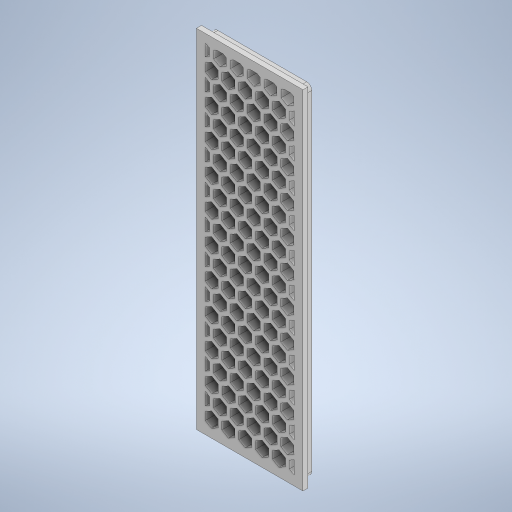
# Autodesk Inventor part: Ventilacion
Saved by Autodesk Inventor 2024 (Build 280153000, 153)
## iProperties
Created: 2023-11-28
Part Number: Ventilacion
Material: Genérico
Document SubType Name: Modeling
Designer: sergi
Density: 1 g/cm^3
Appearance: Valor por defecto
Author: sergi
Autodesk Inventor part; units mm, degrees
(part 1 of 2)
ref_plane "YZ Plane" through (0, 0, 0) normal (1, 0, 0) x (0, 1, 0)
ref_plane "XZ Plane" through (0, 0, 0) normal (0, 1, 0) x (-1, 0, 0)
ref_plane "XY Plane" through (0, 0, 0) normal (0, 0, 1) x (1, 0, 0)
sketch "Boceto1" plane through (0, 0, 0) normal (0, 0, 1) x (1, 0, 0)
  line L0 (-1, 144.7) -> (-1, 9) projected
  line L1 (-1, 9) -> (-41, 9) projected
  line L2 (-41, 9) -> (-41, 144.7) projected
  line L3 (-41, 144.7) -> (-1, 144.7) projected
  line L4 (8, 153.7) -> (-50, 153.7) projected
  line L5 (-50, 0) -> (-50, 153.7) projected
  line L6 (8, 0) -> (-50, 0) projected
  line L7 (8, 153.7) -> (8, 0) projected
  line L8 (-41, 9) -> (-1, 9)
  line L9 (-1, 9) -> (-1, 144.7)
  line L10 (-1, 144.7) -> (-41, 144.7)
  line L11 (-41, 144.7) -> (-41, 9)
  line L12 (-40.65, 144.35) -> (-40.65, 9.35)
  line L13 (-40.65, 9.35) -> (-1.35, 9.35)
  line L14 (-1.35, 9.35) -> (-1.35, 144.35)
  line L15 (-1.35, 144.35) -> (-40.65, 144.35)
  line L16 (-3.35, 11.35) -> (-38.65, 11.35)
  line L17 (-38.65, 11.35) -> (-38.65, 142.35)
  line L18 (-38.65, 142.35) -> (-3.35, 142.35)
  line L19 (-3.35, 142.35) -> (-3.35, 11.35)
  line L20 (-36.1519, 17.25) -> (-33.5538, 15.75)
  line L21 (-33.5538, 15.75) -> (-33.5538, 12.75)
  line L22 (-33.5538, 12.75) -> (-36.1519, 11.25)
  line L23 (-36.1519, 11.25) -> (-38.75, 12.75)
  line L24 (-38.75, 12.75) -> (-38.75, 15.75)
  line L25 (-38.75, 15.75) -> (-36.1519, 17.25)
  line L26 (-38.65, 11.35) -> (-38.65, 12.75)
  line L27 (-30.2058, 21.75) -> (-30.2058, 18.75)
  line L28 (-30.2058, 18.75) -> (-32.8038, 17.25)
  line L29 (-32.8038, 17.25) -> (-35.4019, 18.75)
  line L30 (-35.4019, 18.75) -> (-35.4019, 21.75)
  line L31 (-35.4019, 21.75) -> (-32.8038, 23.25)
  line L32 (-32.8038, 23.25) -> (-30.2058, 21.75)
  line L33 (-26.8577, 15.75) -> (-26.8577, 12.75)
  line L34 (-26.8577, 12.75) -> (-29.4558, 11.25)
  line L35 (-29.4558, 11.25) -> (-32.0538, 12.75)
  line L36 (-32.0538, 12.75) -> (-32.0538, 15.75)
  line L37 (-32.0538, 15.75) -> (-29.4558, 17.25)
  line L38 (-29.4558, 17.25) -> (-26.8577, 15.75)
  line L39 (-28.7058, 18.75) -> (-28.7058, 21.75)
  line L40 (-28.7058, 21.75) -> (-26.1077, 23.25)
  line L41 (-26.1077, 23.25) -> (-23.5096, 21.75)
  line L42 (-23.5096, 21.75) -> (-23.5096, 18.75)
  line L43 (-23.5096, 18.75) -> (-26.1077, 17.25)
  line L44 (-26.1077, 17.25) -> (-28.7058, 18.75)
  line L45 (-22.0096, 18.75) -> (-22.0096, 21.75)
  line L46 (-22.0096, 21.75) -> (-19.4115, 23.25)
  line L47 (-19.4115, 23.25) -> (-16.8135, 21.75)
  line L48 (-16.8135, 21.75) -> (-16.8135, 18.75)
  line L49 (-16.8135, 18.75) -> (-19.4115, 17.25)
  line L50 (-19.4115, 17.25) -> (-22.0096, 18.75)
  line L51 (-15.3135, 18.75) -> (-15.3135, 21.75)
  line L52 (-15.3135, 21.75) -> (-12.7154, 23.25)
  line L53 (-12.7154, 23.25) -> (-10.1173, 21.75)
  line L54 (-10.1173, 21.75) -> (-10.1173, 18.75)
  line L55 (-10.1173, 18.75) -> (-12.7154, 17.25)
  line L56 (-12.7154, 17.25) -> (-15.3135, 18.75)
  line L57 (-8.6173, 18.75) -> (-8.6173, 21.75)
  line L58 (-8.6173, 21.75) -> (-6.0192, 23.25)
  line L59 (-6.0192, 23.25) -> (-3.4212, 21.75)
  line L60 (-3.4212, 21.75) -> (-3.4212, 18.75)
  line L61 (-3.4212, 18.75) -> (-6.0192, 17.25)
  line L62 (-6.0192, 17.25) -> (-8.6173, 18.75)
  line L63 (-40.65, 17.914) -> (-42.0981, 18.75)
  line L64 (-36.9019, 21.75) -> (-36.9019, 18.75)
  line L65 (-42.0981, 18.75) -> (-42.0981, 21.75)
  line L66 (-42.0981, 21.75) -> (-39.5, 23.25)
  line L67 (-38.65, 22.7593) -> (-36.9019, 21.75)
  line L68 (-36.9019, 18.75) -> (-39.5, 17.25)
  line L69 (-30.2058, 33.6998) -> (-30.2058, 30.6998)
  line L70 (-30.2058, 30.6998) -> (-32.8038, 29.1998)
  line L71 (-32.8038, 29.1998) -> (-35.4019, 30.6998)
  line L72 (-35.4019, 30.6998) -> (-35.4019, 33.6998)
  line L73 (-35.4019, 33.6998) -> (-32.8038, 35.1998)
  line L74 (-32.8038, 35.1998) -> (-30.2058, 33.6998)
  line L75 (-28.7058, 30.6998) -> (-28.7058, 33.6998)
  line L76 (-28.7058, 33.6998) -> (-26.1077, 35.1998)
  line L77 (-26.1077, 35.1998) -> (-23.5096, 33.6998)
  line L78 (-23.5096, 33.6998) -> (-23.5096, 30.6998)
  line L79 (-23.5096, 30.6998) -> (-26.1077, 29.1998)
  line L80 (-26.1077, 29.1998) -> (-28.7058, 30.6998)
  line L81 (-19.4115, 29.1998) -> (-22.0096, 30.6998)
  line L82 (-16.8135, 33.6998) -> (-16.8135, 30.6998)
  line L83 (-22.0096, 30.6998) -> (-22.0096, 33.6998)
  line L84 (-22.0096, 33.6998) -> (-19.4115, 35.1998)
  line L85 (-19.4115, 35.1998) -> (-16.8135, 33.6998)
  line L86 (-16.8135, 30.6998) -> (-19.4115, 29.1998)
  line L87 (-12.7154, 29.1998) -> (-15.3135, 30.6998)
  line L88 (-10.1173, 33.6998) -> (-10.1173, 30.6998)
  line L89 (-15.3135, 30.6998) -> (-15.3135, 33.6998)
  line L90 (-15.3135, 33.6998) -> (-12.7154, 35.1998)
  line L91 (-12.7154, 35.1998) -> (-10.1173, 33.6998)
  line L92 (-10.1173, 30.6998) -> (-12.7154, 29.1998)
  line L93 (-6.0192, 29.1998) -> (-8.6173, 30.6998)
  line L94 (-3.4212, 33.6998) -> (-3.4212, 30.6998)
  line L95 (-8.6173, 30.6998) -> (-8.6173, 33.6998)
  line L96 (-8.6173, 33.6998) -> (-6.0192, 35.1998)
  line L97 (-6.0192, 35.1998) -> (-3.4212, 33.6998)
  line L98 (-3.4212, 30.6998) -> (-6.0192, 29.1998)
  line L99 (-42.0981, 30.6998) -> (-42.0981, 33.6998)
  line L100 (-42.0981, 33.6998) -> (-39.5, 35.1998)
  line L101 (-39.5, 29.1998) -> (-42.0981, 30.6998)
  line L102 (-36.9019, 33.6998) -> (-36.9019, 30.6998)
  line L103 (-38.65, 34.709) -> (-36.9019, 33.6998)
  line L104 (-36.9019, 30.6998) -> (-38.65, 29.6905)
  line L105 (-26.8577, 39.6998) -> (-26.8577, 36.6998)
  line L106 (-26.8577, 36.6998) -> (-29.4558, 35.1998)
  line L107 (-29.4558, 35.1998) -> (-32.0538, 36.6998)
  line L108 (-32.0538, 36.6998) -> (-32.0538, 39.6998)
  line L109 (-32.0538, 39.6998) -> (-29.4558, 41.1998)
  line L110 (-29.4558, 41.1998) -> (-26.8577, 39.6998)
  line L111 (-25.3577, 36.6998) -> (-25.3577, 39.6998)
  line L112 (-25.3577, 39.6998) -> (-22.7596, 41.1998)
  line L113 (-22.7596, 41.1998) -> (-20.1615, 39.6998)
  line L114 (-20.1615, 39.6998) -> (-20.1615, 36.6998)
  line L115 (-20.1615, 36.6998) -> (-22.7596, 35.1998)
  line L116 (-22.7596, 35.1998) -> (-25.3577, 36.6998)
  line L117 (-16.0635, 35.1998) -> (-18.6615, 36.6998)
  line L118 (-13.4654, 39.6998) -> (-13.4654, 36.6998)
  line L119 (-18.6615, 36.6998) -> (-18.6615, 39.6998)
  line L120 (-18.6615, 39.6998) -> (-16.0635, 41.1998)
  line L121 (-16.0635, 41.1998) -> (-13.4654, 39.6998)
  line L122 (-13.4654, 36.6998) -> (-16.0635, 35.1998)
  line L123 (-9.3673, 35.1998) -> (-11.9654, 36.6998)
  line L124 (-6.7692, 39.6998) -> (-6.7692, 36.6998)
  line L125 (-11.9654, 36.6998) -> (-11.9654, 39.6998)
  line L126 (-11.9654, 39.6998) -> (-9.3673, 41.1998)
  line L127 (-9.3673, 41.1998) -> (-6.7692, 39.6998)
  line L128 (-6.7692, 36.6998) -> (-9.3673, 35.1998)
  line L129 (-2.6712, 35.1998) -> (-5.2692, 36.6998)
  line L130 (-0.0731, 39.6998) -> (-0.0731, 36.6998)
  line L131 (-5.2692, 36.6998) -> (-5.2692, 39.6998)
  line L132 (-5.2692, 39.6998) -> (-2.6712, 41.1998)
  line L133 (-1.35, 40.437) -> (-0.0731, 39.6998)
  line L134 (-0.0731, 36.6998) -> (-1.35, 35.9625)
  line L135 (-38.75, 36.6998) -> (-38.75, 39.6998)
  line L136 (-38.75, 39.6998) -> (-36.1519, 41.1998)
  line L137 (-36.1519, 35.1998) -> (-38.75, 36.6998)
  line L138 (-33.5538, 39.6998) -> (-33.5538, 36.6998)
  line L139 (-36.1519, 41.1998) -> (-33.5538, 39.6998)
  line L140 (-33.5538, 36.6998) -> (-36.1519, 35.1998)
  line L141 (-30.2058, 45.6998) -> (-30.2058, 42.6998)
  line L142 (-30.2058, 42.6998) -> (-32.8038, 41.1998)
  line L143 (-32.8038, 41.1998) -> (-35.4019, 42.6998)
  line L144 (-35.4019, 42.6998) -> (-35.4019, 45.6998)
  line L145 (-35.4019, 45.6998) -> (-32.8038, 47.1998)
  line L146 (-32.8038, 47.1998) -> (-30.2058, 45.6998)
  line L147 (-28.7058, 42.6998) -> (-28.7058, 45.6998)
  line L148 (-28.7058, 45.6998) -> (-26.1077, 47.1998)
  line L149 (-26.1077, 47.1998) -> (-23.5096, 45.6998)
  line L150 (-23.5096, 45.6998) -> (-23.5096, 42.6998)
  line L151 (-23.5096, 42.6998) -> (-26.1077, 41.1998)
  line L152 (-26.1077, 41.1998) -> (-28.7058, 42.6998)
  line L153 (-19.4115, 41.1998) -> (-22.0096, 42.6998)
  line L154 (-16.8135, 45.6998) -> (-16.8135, 42.6998)
  line L155 (-22.0096, 42.6998) -> (-22.0096, 45.6998)
  line L156 (-22.0096, 45.6998) -> (-19.4115, 47.1998)
  line L157 (-19.4115, 47.1998) -> (-16.8135, 45.6998)
  line L158 (-16.8135, 42.6998) -> (-19.4115, 41.1998)
  line L159 (-12.7154, 41.1998) -> (-15.3135, 42.6998)
  line L160 (-10.1173, 45.6998) -> (-10.1173, 42.6998)
  line L161 (-15.3135, 42.6998) -> (-15.3135, 45.6998)
  line L162 (-15.3135, 45.6998) -> (-12.7154, 47.1998)
  line L163 (-12.7154, 47.1998) -> (-10.1173, 45.6998)
  line L164 (-10.1173, 42.6998) -> (-12.7154, 41.1998)
  line L165 (-6.0192, 41.1998) -> (-8.6173, 42.6998)
  line L166 (-3.4212, 45.6998) -> (-3.4212, 42.6998)
  line L167 (-8.6173, 42.6998) -> (-8.6173, 45.6998)
  line L168 (-8.6173, 45.6998) -> (-6.0192, 47.1998)
  line L169 (-6.0192, 47.1998) -> (-3.4212, 45.6998)
  line L170 (-3.4212, 42.6998) -> (-6.0192, 41.1998)
  line L171 (-42.0981, 42.6998) -> (-42.0981, 45.6998)
  line L172 (-42.0981, 45.6998) -> (-40.65, 46.5358)
  line L173 (-40.65, 41.8637) -> (-42.0981, 42.6998)
  line L174 (-36.9019, 45.6998) -> (-36.9019, 42.6998)
  line L175 (-39.5, 47.1998) -> (-36.9019, 45.6998)
  line L176 (-36.9019, 42.6998) -> (-39.5, 41.1998)
  line L177 (-26.8577, 51.6998) -> (-26.8577, 48.6998)
  line L178 (-26.8577, 48.6998) -> (-29.4558, 47.1998)
  line L179 (-29.4558, 47.1998) -> (-32.0538, 48.6998)
  line L180 (-32.0538, 48.6998) -> (-32.0538, 51.6998)
  line L181 (-32.0538, 51.6998) -> (-29.4558, 53.1998)
  line L182 (-29.4558, 53.1998) -> (-26.8577, 51.6998)
  line L183 (-25.3577, 48.6998) -> (-25.3577, 51.6998)
  line L184 (-25.3577, 51.6998) -> (-22.7596, 53.1998)
  line L185 (-22.7596, 53.1998) -> (-20.1615, 51.6998)
  line L186 (-20.1615, 51.6998) -> (-20.1615, 48.6998)
  line L187 (-20.1615, 48.6998) -> (-22.7596, 47.1998)
  line L188 (-22.7596, 47.1998) -> (-25.3577, 48.6998)
  line L189 (-16.0635, 47.1998) -> (-18.6615, 48.6998)
  line L190 (-13.4654, 51.6998) -> (-13.4654, 48.6998)
  line L191 (-18.6615, 48.6998) -> (-18.6615, 51.6998)
  line L192 (-18.6615, 51.6998) -> (-16.0635, 53.1998)
  line L193 (-16.0635, 53.1998) -> (-13.4654, 51.6998)
  line L194 (-13.4654, 48.6998) -> (-16.0635, 47.1998)
  line L195 (-9.3673, 47.1998) -> (-11.9654, 48.6998)
  line L196 (-6.7692, 51.6998) -> (-6.7692, 48.6998)
  line L197 (-11.9654, 48.6998) -> (-11.9654, 51.6998)
  line L198 (-11.9654, 51.6998) -> (-9.3673, 53.1998)
  line L199 (-9.3673, 53.1998) -> (-6.7692, 51.6998)
  line L200 (-6.7692, 48.6998) -> (-9.3673, 47.1998)
  line L201 (-2.6712, 47.1998) -> (-5.2692, 48.6998)
  line L202 (-0.0731, 51.6998) -> (-0.0731, 48.6998)
  line L203 (-5.2692, 48.6998) -> (-5.2692, 51.6998)
  line L204 (-5.2692, 51.6998) -> (-2.6712, 53.1998)
  line L205 (-1.35, 52.437) -> (-0.0731, 51.6998)
  line L206 (-0.0731, 48.6998) -> (-1.35, 47.9625)
  line L207 (-38.75, 48.6998) -> (-38.75, 51.6998)
  line L208 (-38.75, 51.6998) -> (-36.1519, 53.1998)
  line L209 (-36.1519, 47.1998) -> (-38.75, 48.6998)
  line L210 (-33.5538, 51.6998) -> (-33.5538, 48.6998)
  line L211 (-36.1519, 53.1998) -> (-33.5538, 51.6998)
  line L212 (-33.5538, 48.6998) -> (-36.1519, 47.1998)
  line L213 (-30.2058, 57.6998) -> (-30.2058, 54.6998)
  line L214 (-30.2058, 54.6998) -> (-32.8038, 53.1998)
  line L215 (-32.8038, 53.1998) -> (-35.4019, 54.6998)
  line L216 (-35.4019, 54.6998) -> (-35.4019, 57.6998)
  line L217 (-35.4019, 57.6998) -> (-32.8038, 59.1998)
  line L218 (-32.8038, 59.1998) -> (-30.2058, 57.6998)
  line L219 (-28.7058, 54.6998) -> (-28.7058, 57.6998)
  line L220 (-28.7058, 57.6998) -> (-26.1077, 59.1998)
  line L221 (-26.1077, 59.1998) -> (-23.5096, 57.6998)
  line L222 (-23.5096, 57.6998) -> (-23.5096, 54.6998)
  line L223 (-23.5096, 54.6998) -> (-26.1077, 53.1998)
  line L224 (-26.1077, 53.1998) -> (-28.7058, 54.6998)
  line L225 (-19.4115, 53.1998) -> (-22.0096, 54.6998)
  line L226 (-16.8135, 57.6998) -> (-16.8135, 54.6998)
  line L227 (-22.0096, 54.6998) -> (-22.0096, 57.6998)
  line L228 (-22.0096, 57.6998) -> (-19.4115, 59.1998)
  line L229 (-19.4115, 59.1998) -> (-16.8135, 57.6998)
  line L230 (-16.8135, 54.6998) -> (-19.4115, 53.1998)
  line L231 (-12.7154, 53.1998) -> (-15.3135, 54.6998)
  line L232 (-10.1173, 57.6998) -> (-10.1173, 54.6998)
  line L233 (-15.3135, 54.6998) -> (-15.3135, 57.6998)
  line L234 (-15.3135, 57.6998) -> (-12.7154, 59.1998)
  line L235 (-12.7154, 59.1998) -> (-10.1173, 57.6998)
  line L236 (-10.1173, 54.6998) -> (-12.7154, 53.1998)
  line L237 (-6.0192, 53.1998) -> (-8.6173, 54.6998)
  line L238 (-3.4212, 57.6998) -> (-3.4212, 54.6998)
  line L239 (-8.6173, 54.6998) -> (-8.6173, 57.6998)
  line L240 (-8.6173, 57.6998) -> (-6.0192, 59.1998)
  line L241 (-6.0192, 59.1998) -> (-3.4212, 57.6998)
  line L242 (-3.4212, 54.6998) -> (-6.0192, 53.1998)
  line L243 (-42.0981, 54.6998) -> (-42.0981, 57.6998)
  line L244 (-42.0981, 57.6998) -> (-40.65, 58.5358)
  line L245 (-40.65, 53.8637) -> (-42.0981, 54.6998)
  line L246 (-36.9019, 57.6998) -> (-36.9019, 54.6998)
  line L247 (-39.5, 59.1998) -> (-36.9019, 57.6998)
  line L248 (-36.9019, 54.6998) -> (-39.5, 53.1998)
  line L249 (-26.8577, 63.6998) -> (-26.8577, 60.6998)
  line L250 (-26.8577, 60.6998) -> (-29.4558, 59.1998)
  line L251 (-29.4558, 59.1998) -> (-32.0538, 60.6998)
  line L252 (-32.0538, 60.6998) -> (-32.0538, 63.6998)
  line L253 (-32.0538, 63.6998) -> (-29.4558, 65.1998)
  line L254 (-29.4558, 65.1998) -> (-26.8577, 63.6998)
  line L255 (-25.3577, 60.6998) -> (-25.3577, 63.6998)
  line L256 (-25.3577, 63.6998) -> (-22.7596, 65.1998)
  line L257 (-22.7596, 65.1998) -> (-20.1615, 63.6998)
  line L258 (-20.1615, 63.6998) -> (-20.1615, 60.6998)
  line L259 (-20.1615, 60.6998) -> (-22.7596, 59.1998)
  line L260 (-22.7596, 59.1998) -> (-25.3577, 60.6998)
  line L261 (-16.0635, 59.1998) -> (-18.6615, 60.6998)
  line L262 (-13.4654, 63.6998) -> (-13.4654, 60.6998)
  line L263 (-18.6615, 60.6998) -> (-18.6615, 63.6998)
  line L264 (-18.6615, 63.6998) -> (-16.0635, 65.1998)
  line L265 (-16.0635, 65.1998) -> (-13.4654, 63.6998)
  line L266 (-13.4654, 60.6998) -> (-16.0635, 59.1998)
  line L267 (-9.3673, 59.1998) -> (-11.9654, 60.6998)
  line L268 (-6.7692, 63.6998) -> (-6.7692, 60.6998)
  line L269 (-11.9654, 60.6998) -> (-11.9654, 63.6998)
  line L270 (-11.9654, 63.6998) -> (-9.3673, 65.1998)
  line L271 (-9.3673, 65.1998) -> (-6.7692, 63.6998)
  line L272 (-6.7692, 60.6998) -> (-9.3673, 59.1998)
  line L273 (-2.6712, 59.1998) -> (-5.2692, 60.6998)
  line L274 (-0.0731, 63.6998) -> (-0.0731, 60.6998)
  line L275 (-5.2692, 60.6998) -> (-5.2692, 63.6998)
  line L276 (-5.2692, 63.6998) -> (-2.6712, 65.1998)
  line L277 (-1.35, 64.437) -> (-0.0731, 63.6998)
  line L278 (-0.0731, 60.6998) -> (-1.35, 59.9625)
  line L279 (-38.75, 60.6998) -> (-38.75, 63.6998)
  line L280 (-38.75, 63.6998) -> (-36.1519, 65.1998)
  line L281 (-36.1519, 59.1998) -> (-38.75, 60.6998)
  line L282 (-33.5538, 63.6998) -> (-33.5538, 60.6998)
  line L283 (-36.1519, 65.1998) -> (-33.5538, 63.6998)
  line L284 (-33.5538, 60.6998) -> (-36.1519, 59.1998)
  line L285 (-30.2058, 69.6998) -> (-30.2058, 66.6998)
  line L286 (-30.2058, 66.6998) -> (-32.8038, 65.1998)
  line L287 (-32.8038, 65.1998) -> (-35.4019, 66.6998)
  line L288 (-35.4019, 66.6998) -> (-35.4019, 69.6998)
  line L289 (-35.4019, 69.6998) -> (-32.8038, 71.1998)
  line L290 (-32.8038, 71.1998) -> (-30.2058, 69.6998)
  line L291 (-28.7058, 66.6998) -> (-28.7058, 69.6998)
  line L292 (-28.7058, 69.6998) -> (-26.1077, 71.1998)
  line L293 (-26.1077, 71.1998) -> (-23.5096, 69.6998)
  line L294 (-23.5096, 69.6998) -> (-23.5096, 66.6998)
  line L295 (-23.5096, 66.6998) -> (-26.1077, 65.1998)
  line L296 (-26.1077, 65.1998) -> (-28.7058, 66.6998)
  line L297 (-19.4115, 65.1998) -> (-22.0096, 66.6998)
  line L298 (-16.8135, 69.6998) -> (-16.8135, 66.6998)
  line L299 (-22.0096, 66.6998) -> (-22.0096, 69.6998)
  line L300 (-22.0096, 69.6998) -> (-19.4115, 71.1998)
  line L301 (-19.4115, 71.1998) -> (-16.8135, 69.6998)
  line L302 (-16.8135, 66.6998) -> (-19.4115, 65.1998)
  line L303 (-12.7154, 65.1998) -> (-15.3135, 66.6998)
  line L304 (-10.1173, 69.6998) -> (-10.1173, 66.6998)
  line L305 (-15.3135, 66.6998) -> (-15.3135, 69.6998)
  line L306 (-15.3135, 69.6998) -> (-12.7154, 71.1998)
  line L307 (-12.7154, 71.1998) -> (-10.1173, 69.6998)
  line L308 (-10.1173, 66.6998) -> (-12.7154, 65.1998)
  line L309 (-6.0192, 65.1998) -> (-8.6173, 66.6998)
  line L310 (-3.4212, 69.6998) -> (-3.4212, 66.6998)
  line L311 (-8.6173, 66.6998) -> (-8.6173, 69.6998)
  line L312 (-8.6173, 69.6998) -> (-6.0192, 71.1998)
  line L313 (-6.0192, 71.1998) -> (-3.4212, 69.6998)
  line L314 (-3.4212, 66.6998) -> (-6.0192, 65.1998)
  line L315 (-42.0981, 66.6998) -> (-42.0981, 69.6998)
  line L316 (-42.0981, 69.6998) -> (-40.65, 70.5358)
  line L317 (-40.65, 65.8637) -> (-42.0981, 66.6998)
  line L318 (-36.9019, 69.6998) -> (-36.9019, 66.6998)
  line L319 (-39.5, 71.1998) -> (-36.9019, 69.6998)
  line L320 (-36.9019, 66.6998) -> (-39.5, 65.1998)
  line L321 (-26.8577, 75.6998) -> (-26.8577, 72.6998)
  line L322 (-26.8577, 72.6998) -> (-29.4558, 71.1998)
  line L323 (-29.4558, 71.1998) -> (-32.0538, 72.6998)
  line L324 (-32.0538, 72.6998) -> (-32.0538, 75.6998)
  line L325 (-32.0538, 75.6998) -> (-29.4558, 77.1998)
  line L326 (-29.4558, 77.1998) -> (-26.8577, 75.6998)
  line L327 (-25.3577, 72.6998) -> (-25.3577, 75.6998)
  line L328 (-25.3577, 75.6998) -> (-22.7596, 77.1998)
  line L329 (-22.7596, 77.1998) -> (-20.1615, 75.6998)
  line L330 (-20.1615, 75.6998) -> (-20.1615, 72.6998)
  line L331 (-20.1615, 72.6998) -> (-22.7596, 71.1998)
  line L332 (-22.7596, 71.1998) -> (-25.3577, 72.6998)
  line L333 (-16.0635, 71.1998) -> (-18.6615, 72.6998)
  line L334 (-13.4654, 75.6998) -> (-13.4654, 72.6998)
  line L335 (-18.6615, 72.6998) -> (-18.6615, 75.6998)
  line L336 (-18.6615, 75.6998) -> (-16.0635, 77.1998)
  line L337 (-16.0635, 77.1998) -> (-13.4654, 75.6998)
  line L338 (-13.4654, 72.6998) -> (-16.0635, 71.1998)
  line L339 (-9.3673, 71.1998) -> (-11.9654, 72.6998)
  line L340 (-6.7692, 75.6998) -> (-6.7692, 72.6998)
  line L341 (-11.9654, 72.6998) -> (-11.9654, 75.6998)
  line L342 (-11.9654, 75.6998) -> (-9.3673, 77.1998)
  line L343 (-9.3673, 77.1998) -> (-6.7692, 75.6998)
  line L344 (-6.7692, 72.6998) -> (-9.3673, 71.1998)
  line L345 (-2.6712, 71.1998) -> (-5.2692, 72.6998)
  line L346 (-0.0731, 75.6998) -> (-0.0731, 72.6998)
  line L347 (-5.2692, 72.6998) -> (-5.2692, 75.6998)
  line L348 (-5.2692, 75.6998) -> (-2.6712, 77.1998)
  line L349 (-1.35, 76.437) -> (-0.0731, 75.6998)
  line L350 (-0.0731, 72.6998) -> (-1.35, 71.9625)
  line L351 (-38.75, 72.6998) -> (-38.75, 75.6998)
  line L352 (-38.75, 75.6998) -> (-36.1519, 77.1998)
  line L353 (-36.1519, 71.1998) -> (-38.75, 72.6998)
  line L354 (-33.5538, 75.6998) -> (-33.5538, 72.6998)
  line L355 (-36.1519, 77.1998) -> (-33.5538, 75.6998)
  line L356 (-33.5538, 72.6998) -> (-36.1519, 71.1998)
  line L357 (-30.2058, 81.6998) -> (-30.2058, 78.6998)
  line L358 (-30.2058, 78.6998) -> (-32.8038, 77.1998)
  line L359 (-32.8038, 77.1998) -> (-35.4019, 78.6998)
  line L360 (-35.4019, 78.6998) -> (-35.4019, 81.6998)
  line L361 (-35.4019, 81.6998) -> (-32.8038, 83.1998)
  line L362 (-32.8038, 83.1998) -> (-30.2058, 81.6998)
  line L363 (-28.7058, 78.6998) -> (-28.7058, 81.6998)
  line L364 (-28.7058, 81.6998) -> (-26.1077, 83.1998)
  line L365 (-26.1077, 83.1998) -> (-23.5096, 81.6998)
  line L366 (-23.5096, 81.6998) -> (-23.5096, 78.6998)
  line L367 (-23.5096, 78.6998) -> (-26.1077, 77.1998)
  line L368 (-26.1077, 77.1998) -> (-28.7058, 78.6998)
  line L369 (-19.4115, 77.1998) -> (-22.0096, 78.6998)
  line L370 (-16.8135, 81.6998) -> (-16.8135, 78.6998)
  line L371 (-22.0096, 78.6998) -> (-22.0096, 81.6998)
  line L372 (-22.0096, 81.6998) -> (-19.4115, 83.1998)
  line L373 (-19.4115, 83.1998) -> (-16.8135, 81.6998)
  line L374 (-16.8135, 78.6998) -> (-19.4115, 77.1998)
  line L375 (-12.7154, 77.1998) -> (-15.3135, 78.6998)
  line L376 (-10.1173, 81.6998) -> (-10.1173, 78.6998)
  line L377 (-15.3135, 78.6998) -> (-15.3135, 81.6998)
  line L378 (-15.3135, 81.6998) -> (-12.7154, 83.1998)
  line L379 (-12.7154, 83.1998) -> (-10.1173, 81.6998)
  line L380 (-10.1173, 78.6998) -> (-12.7154, 77.1998)
  line L381 (-6.0192, 77.1998) -> (-8.6173, 78.6998)
  line L382 (-3.4212, 81.6998) -> (-3.4212, 78.6998)
  line L383 (-8.6173, 78.6998) -> (-8.6173, 81.6998)
  line L384 (-8.6173, 81.6998) -> (-6.0192, 83.1998)
  line L385 (-6.0192, 83.1998) -> (-3.4212, 81.6998)
  line L386 (-3.4212, 78.6998) -> (-6.0192, 77.1998)
  line L387 (-42.0981, 78.6998) -> (-42.0981, 81.6998)
  line L388 (-42.0981, 81.6998) -> (-40.65, 82.5358)
  line L389 (-40.65, 77.8637) -> (-42.0981, 78.6998)
  line L390 (-36.9019, 81.6998) -> (-36.9019, 78.6998)
  line L391 (-39.5, 83.1998) -> (-36.9019, 81.6998)
  line L392 (-36.9019, 78.6998) -> (-39.5, 77.1998)
  line L393 (-26.8577, 87.6998) -> (-26.8577, 84.6998)
  line L394 (-26.8577, 84.6998) -> (-29.4558, 83.1998)
  line L395 (-29.4558, 83.1998) -> (-32.0538, 84.6998)
  line L396 (-32.0538, 84.6998) -> (-32.0538, 87.6998)
  line L397 (-32.0538, 87.6998) -> (-29.4558, 89.1998)
  line L398 (-29.4558, 89.1998) -> (-26.8577, 87.6998)
  line L399 (-25.3577, 84.6998) -> (-25.3577, 87.6998)
  line L400 (-25.3577, 87.6998) -> (-22.7596, 89.1998)
  line L401 (-22.7596, 89.1998) -> (-20.1615, 87.6998)
  line L402 (-20.1615, 87.6998) -> (-20.1615, 84.6998)
  line L403 (-20.1615, 84.6998) -> (-22.7596, 83.1998)
  line L404 (-22.7596, 83.1998) -> (-25.3577, 84.6998)
  line L405 (-16.0635, 83.1998) -> (-18.6615, 84.6998)
  line L406 (-13.4654, 87.6998) -> (-13.4654, 84.6998)
  line L407 (-18.6615, 84.6998) -> (-18.6615, 87.6998)
  line L408 (-18.6615, 87.6998) -> (-16.0635, 89.1998)
  line L409 (-16.0635, 89.1998) -> (-13.4654, 87.6998)
  line L410 (-13.4654, 84.6998) -> (-16.0635, 83.1998)
  line L411 (-9.3673, 83.1998) -> (-11.9654, 84.6998)
  line L412 (-6.7692, 87.6998) -> (-6.7692, 84.6998)
  line L413 (-11.9654, 84.6998) -> (-11.9654, 87.6998)
  line L414 (-11.9654, 87.6998) -> (-9.3673, 89.1998)
  line L415 (-9.3673, 89.1998) -> (-6.7692, 87.6998)
  line L416 (-6.7692, 84.6998) -> (-9.3673, 83.1998)
  line L417 (-2.6712, 83.1998) -> (-5.2692, 84.6998)
  line L418 (-0.0731, 87.6998) -> (-0.0731, 84.6998)
  line L419 (-5.2692, 84.6998) -> (-5.2692, 87.6998)
  line L420 (-5.2692, 87.6998) -> (-2.6712, 89.1998)
  line L421 (-1.35, 88.437) -> (-0.0731, 87.6998)
  line L422 (-0.0731, 84.6998) -> (-1.35, 83.9625)
  line L423 (-38.75, 84.6998) -> (-38.75, 87.6998)
  line L424 (-38.75, 87.6998) -> (-36.1519, 89.1998)
  line L425 (-36.1519, 83.1998) -> (-38.75, 84.6998)
  line L426 (-33.5538, 87.6998) -> (-33.5538, 84.6998)
  line L427 (-36.1519, 89.1998) -> (-33.5538, 87.6998)
  line L428 (-33.5538, 84.6998) -> (-36.1519, 83.1998)
  line L429 (-30.2058, 93.6998) -> (-30.2058, 90.6998)
  line L430 (-30.2058, 90.6998) -> (-32.8038, 89.1998)
  line L431 (-32.8038, 89.1998) -> (-35.4019, 90.6998)
  line L432 (-35.4019, 90.6998) -> (-35.4019, 93.6998)
  line L433 (-35.4019, 93.6998) -> (-32.8038, 95.1998)
  line L434 (-32.8038, 95.1998) -> (-30.2058, 93.6998)
  line L435 (-28.7058, 90.6998) -> (-28.7058, 93.6998)
  line L436 (-28.7058, 93.6998) -> (-26.1077, 95.1998)
  line L437 (-26.1077, 95.1998) -> (-23.5096, 93.6998)
  line L438 (-23.5096, 93.6998) -> (-23.5096, 90.6998)
  line L439 (-23.5096, 90.6998) -> (-26.1077, 89.1998)
  line L440 (-26.1077, 89.1998) -> (-28.7058, 90.6998)
  line L441 (-19.4115, 89.1998) -> (-22.0096, 90.6998)
  line L442 (-16.8135, 93.6998) -> (-16.8135, 90.6998)
  line L443 (-22.0096, 90.6998) -> (-22.0096, 93.6998)
  line L444 (-22.0096, 93.6998) -> (-19.4115, 95.1998)
  line L445 (-19.4115, 95.1998) -> (-16.8135, 93.6998)
  line L446 (-16.8135, 90.6998) -> (-19.4115, 89.1998)
  line L447 (-12.7154, 89.1998) -> (-15.3135, 90.6998)
  line L448 (-10.1173, 93.6998) -> (-10.1173, 90.6998)
  line L449 (-15.3135, 90.6998) -> (-15.3135, 93.6998)
  line L450 (-15.3135, 93.6998) -> (-12.7154, 95.1998)
  line L451 (-12.7154, 95.1998) -> (-10.1173, 93.6998)
  line L452 (-10.1173, 90.6998) -> (-12.7154, 89.1998)
  line L453 (-6.0192, 89.1998) -> (-8.6173, 90.6998)
  line L454 (-3.4212, 93.6998) -> (-3.4212, 90.6998)
  line L455 (-8.6173, 90.6998) -> (-8.6173, 93.6998)
  line L456 (-8.6173, 93.6998) -> (-6.0192, 95.1998)
  line L457 (-6.0192, 95.1998) -> (-3.4212, 93.6998)
  line L458 (-3.4212, 90.6998) -> (-6.0192, 89.1998)
  line L459 (-42.0981, 90.6998) -> (-42.0981, 93.6998)
  line L460 (-42.0981, 93.6998) -> (-40.65, 94.5358)
  line L461 (-40.65, 89.8637) -> (-42.0981, 90.6998)
  line L462 (-36.9019, 93.6998) -> (-36.9019, 90.6998)
  line L463 (-39.5, 95.1998) -> (-36.9019, 93.6998)
  line L464 (-36.9019, 90.6998) -> (-39.5, 89.1998)
  line L465 (-26.8577, 99.6998) -> (-26.8577, 96.6998)
  line L466 (-26.8577, 96.6998) -> (-29.4558, 95.1998)
  line L467 (-29.4558, 95.1998) -> (-32.0538, 96.6998)
  line L468 (-32.0538, 96.6998) -> (-32.0538, 99.6998)
  line L469 (-32.0538, 99.6998) -> (-29.4558, 101.1998)
  line L470 (-29.4558, 101.1998) -> (-26.8577, 99.6998)
  line L471 (-25.3577, 96.6998) -> (-25.3577, 99.6998)
  line L472 (-25.3577, 99.6998) -> (-22.7596, 101.1998)
  line L473 (-22.7596, 101.1998) -> (-20.1615, 99.6998)
  line L474 (-20.1615, 99.6998) -> (-20.1615, 96.6998)
  line L475 (-20.1615, 96.6998) -> (-22.7596, 95.1998)
  line L476 (-22.7596, 95.1998) -> (-25.3577, 96.6998)
  line L477 (-16.0635, 95.1998) -> (-18.6615, 96.6998)
  line L478 (-13.4654, 99.6998) -> (-13.4654, 96.6998)
  line L479 (-18.6615, 96.6998) -> (-18.6615, 99.6998)
  line L480 (-18.6615, 99.6998) -> (-16.0635, 101.1998)
  line L481 (-16.0635, 101.1998) -> (-13.4654, 99.6998)
  line L482 (-13.4654, 96.6998) -> (-16.0635, 95.1998)
  line L483 (-9.3673, 95.1998) -> (-11.9654, 96.6998)
  line L484 (-6.7692, 99.6998) -> (-6.7692, 96.6998)
  line L485 (-11.9654, 96.6998) -> (-11.9654, 99.6998)
  line L486 (-11.9654, 99.6998) -> (-9.3673, 101.1998)
  line L487 (-9.3673, 101.1998) -> (-6.7692, 99.6998)
  line L488 (-6.7692, 96.6998) -> (-9.3673, 95.1998)
  line L489 (-2.6712, 95.1998) -> (-5.2692, 96.6998)
  line L490 (-0.0731, 99.6998) -> (-0.0731, 96.6998)
  line L491 (-5.2692, 96.6998) -> (-5.2692, 99.6998)
  line L492 (-5.2692, 99.6998) -> (-2.6712, 101.1998)
  line L493 (-1.35, 100.437) -> (-0.0731, 99.6998)
  line L494 (-0.0731, 96.6998) -> (-1.35, 95.9625)
  line L495 (-38.75, 96.6998) -> (-38.75, 99.6998)
  line L496 (-38.75, 99.6998) -> (-36.1519, 101.1998)
  line L497 (-36.1519, 95.1998) -> (-38.75, 96.6998)
  line L498 (-33.5538, 99.6998) -> (-33.5538, 96.6998)
  line L499 (-36.1519, 101.1998) -> (-33.5538, 99.6998)
  line L500 (-33.5538, 96.6998) -> (-36.1519, 95.1998)
  line L501 (-30.2058, 105.6998) -> (-30.2058, 102.6998)
  line L502 (-30.2058, 102.6998) -> (-32.8038, 101.1998)
  line L503 (-32.8038, 101.1998) -> (-35.4019, 102.6998)
  line L504 (-35.4019, 102.6998) -> (-35.4019, 105.6998)
  line L505 (-35.4019, 105.6998) -> (-32.8038, 107.1998)
  line L506 (-32.8038, 107.1998) -> (-30.2058, 105.6998)
  line L507 (-28.7058, 102.6998) -> (-28.7058, 105.6998)
  line L508 (-28.7058, 105.6998) -> (-26.1077, 107.1998)
  line L509 (-26.1077, 107.1998) -> (-23.5096, 105.6998)
  line L510 (-23.5096, 105.6998) -> (-23.5096, 102.6998)
  line L511 (-23.5096, 102.6998) -> (-26.1077, 101.1998)
  line L512 (-26.1077, 101.1998) -> (-28.7058, 102.6998)
  line L513 (-19.4115, 101.1998) -> (-22.0096, 102.6998)
  line L514 (-16.8135, 105.6998) -> (-16.8135, 102.6998)
  line L515 (-22.0096, 102.6998) -> (-22.0096, 105.6998)
  line L516 (-22.0096, 105.6998) -> (-19.4115, 107.1998)
  line L517 (-19.4115, 107.1998) -> (-16.8135, 105.6998)
  line L518 (-16.8135, 102.6998) -> (-19.4115, 101.1998)
  line L519 (-12.7154, 101.1998) -> (-15.3135, 102.6998)
  line L520 (-10.1173, 105.6998) -> (-10.1173, 102.6998)
  line L521 (-15.3135, 102.6998) -> (-15.3135, 105.6998)
  line L522 (-15.3135, 105.6998) -> (-12.7154, 107.1998)
  line L523 (-12.7154, 107.1998) -> (-10.1173, 105.6998)
  line L524 (-10.1173, 102.6998) -> (-12.7154, 101.1998)
  line L525 (-6.0192, 101.1998) -> (-8.6173, 102.6998)
  line L526 (-3.4212, 105.6998) -> (-3.4212, 102.6998)
  line L527 (-8.6173, 102.6998) -> (-8.6173, 105.6998)
  line L528 (-8.6173, 105.6998) -> (-6.0192, 107.1998)
  line L529 (-6.0192, 107.1998) -> (-3.4212, 105.6998)
  line L530 (-3.4212, 102.6998) -> (-6.0192, 101.1998)
  line L531 (-42.0981, 102.6998) -> (-42.0981, 105.6998)
  line L532 (-42.0981, 105.6998) -> (-40.65, 106.5358)
  line L533 (-40.65, 101.8637) -> (-42.0981, 102.6998)
  line L534 (-36.9019, 105.6998) -> (-36.9019, 102.6998)
  line L535 (-39.5, 107.1998) -> (-36.9019, 105.6998)
  line L536 (-36.9019, 102.6998) -> (-39.5, 101.1998)
  line L537 (-26.8577, 111.6998) -> (-26.8577, 108.6998)
  line L538 (-26.8577, 108.6998) -> (-29.4558, 107.1998)
  line L539 (-29.4558, 107.1998) -> (-32.0538, 108.6998)
  line L540 (-32.0538, 108.6998) -> (-32.0538, 111.6998)
  line L541 (-32.0538, 111.6998) -> (-29.4558, 113.1998)
  line L542 (-29.4558, 113.1998) -> (-26.8577, 111.6998)
  line L543 (-25.3577, 108.6998) -> (-25.3577, 111.6998)
  line L544 (-25.3577, 111.6998) -> (-22.7596, 113.1998)
  line L545 (-22.7596, 113.1998) -> (-20.1615, 111.6998)
  line L546 (-20.1615, 111.6998) -> (-20.1615, 108.6998)
  line L547 (-20.1615, 108.6998) -> (-22.7596, 107.1998)
  line L548 (-22.7596, 107.1998) -> (-25.3577, 108.6998)
  line L549 (-16.0635, 107.1998) -> (-18.6615, 108.6998)
  line L550 (-13.4654, 111.6998) -> (-13.4654, 108.6998)
  line L551 (-18.6615, 108.6998) -> (-18.6615, 111.6998)
  line L552 (-18.6615, 111.6998) -> (-16.0635, 113.1998)
  line L553 (-16.0635, 113.1998) -> (-13.4654, 111.6998)
  line L554 (-13.4654, 108.6998) -> (-16.0635, 107.1998)
  line L555 (-9.3673, 107.1998) -> (-11.9654, 108.6998)
  line L556 (-6.7692, 111.6998) -> (-6.7692, 108.6998)
  line L557 (-11.9654, 108.6998) -> (-11.9654, 111.6998)
  line L558 (-11.9654, 111.6998) -> (-9.3673, 113.1998)
  line L559 (-9.3673, 113.1998) -> (-6.7692, 111.6998)
  line L560 (-6.7692, 108.6998) -> (-9.3673, 107.1998)
  line L561 (-2.6712, 107.1998) -> (-5.2692, 108.6998)
  line L562 (-0.0731, 111.6998) -> (-0.0731, 108.6998)
  line L563 (-5.2692, 108.6998) -> (-5.2692, 111.6998)
  line L564 (-5.2692, 111.6998) -> (-2.6712, 113.1998)
  line L565 (-1.35, 112.437) -> (-0.0731, 111.6998)
  line L566 (-0.0731, 108.6998) -> (-1.35, 107.9625)
  line L567 (-38.75, 108.6998) -> (-38.75, 111.6998)
  line L568 (-38.75, 111.6998) -> (-36.1519, 113.1998)
  line L569 (-36.1519, 107.1998) -> (-38.75, 108.6998)
  line L570 (-33.5538, 111.6998) -> (-33.5538, 108.6998)
  line L571 (-36.1519, 113.1998) -> (-33.5538, 111.6998)
  line L572 (-33.5538, 108.6998) -> (-36.1519, 107.1998)
  line L573 (-30.2058, 117.6998) -> (-30.2058, 114.6998)
  line L574 (-30.2058, 114.6998) -> (-32.8038, 113.1998)
  line L575 (-32.8038, 113.1998) -> (-35.4019, 114.6998)
  line L576 (-35.4019, 114.6998) -> (-35.4019, 117.6998)
  line L577 (-35.4019, 117.6998) -> (-32.8038, 119.1998)
  line L578 (-32.8038, 119.1998) -> (-30.2058, 117.6998)
  line L579 (-28.7058, 114.6998) -> (-28.7058, 117.6998)
  line L580 (-28.7058, 117.6998) -> (-26.1077, 119.1998)
  line L581 (-26.1077, 119.1998) -> (-23.5096, 117.6998)
  line L582 (-23.5096, 117.6998) -> (-23.5096, 114.6998)
  line L583 (-23.5096, 114.6998) -> (-26.1077, 113.1998)
  line L584 (-26.1077, 113.1998) -> (-28.7058, 114.6998)
  line L585 (-19.4115, 113.1998) -> (-22.0096, 114.6998)
  line L586 (-16.8135, 117.6998) -> (-16.8135, 114.6998)
  line L587 (-22.0096, 114.6998) -> (-22.0096, 117.6998)
  line L588 (-22.0096, 117.6998) -> (-19.4115, 119.1998)
  line L589 (-19.4115, 119.1998) -> (-16.8135, 117.6998)
  line L590 (-16.8135, 114.6998) -> (-19.4115, 113.1998)
  line L591 (-12.7154, 113.1998) -> (-15.3135, 114.6998)
  line L592 (-10.1173, 117.6998) -> (-10.1173, 114.6998)
  line L593 (-15.3135, 114.6998) -> (-15.3135, 117.6998)
  line L594 (-15.3135, 117.6998) -> (-12.7154, 119.1998)
  line L595 (-12.7154, 119.1998) -> (-10.1173, 117.6998)
  line L596 (-10.1173, 114.6998) -> (-12.7154, 113.1998)
  line L597 (-6.0192, 113.1998) -> (-8.6173, 114.6998)
  line L598 (-3.4212, 117.6998) -> (-3.4212, 114.6998)
  line L599 (-8.6173, 114.6998) -> (-8.6173, 117.6998)
  line L600 (-8.6173, 117.6998) -> (-6.0192, 119.1998)
  line L601 (-6.0192, 119.1998) -> (-3.4212, 117.6998)
  line L602 (-3.4212, 114.6998) -> (-6.0192, 113.1998)
  line L603 (-42.0981, 114.6998) -> (-42.0981, 117.6998)
  line L604 (-42.0981, 117.6998) -> (-39.5, 119.1998)
  line L605 (-39.5, 113.1998) -> (-42.0981, 114.6998)
  line L606 (-36.9019, 117.6998) -> (-36.9019, 114.6998)
  line L607 (-39.5, 119.1998) -> (-36.9019, 117.6998)
  line L608 (-36.9019, 114.6998) -> (-39.5, 113.1998)
  line L609 (-26.8577, 123.6998) -> (-26.8577, 120.6998)
  line L610 (-26.8577, 120.6998) -> (-29.4558, 119.1998)
  line L611 (-29.4558, 119.1998) -> (-32.0538, 120.6998)
  line L612 (-32.0538, 120.6998) -> (-32.0538, 123.6998)
  line L613 (-32.0538, 123.6998) -> (-29.4558, 125.1998)
  line L614 (-29.4558, 125.1998) -> (-26.8577, 123.6998)
  line L615 (-25.3577, 120.6998) -> (-25.3577, 123.6998)
  line L616 (-25.3577, 123.6998) -> (-22.7596, 125.1998)
  line L617 (-22.7596, 125.1998) -> (-20.1615, 123.6998)
  line L618 (-20.1615, 123.6998) -> (-20.1615, 120.6998)
  line L619 (-20.1615, 120.6998) -> (-22.7596, 119.1998)
  line L620 (-22.7596, 119.1998) -> (-25.3577, 120.6998)
  line L621 (-16.0635, 119.1998) -> (-18.6615, 120.6998)
  line L622 (-13.4654, 123.6998) -> (-13.4654, 120.6998)
  line L623 (-18.6615, 120.6998) -> (-18.6615, 123.6998)
  line L624 (-18.6615, 123.6998) -> (-16.0635, 125.1998)
  line L625 (-16.0635, 125.1998) -> (-13.4654, 123.6998)
  line L626 (-13.4654, 120.6998) -> (-16.0635, 119.1998)
  line L627 (-9.3673, 119.1998) -> (-11.9654, 120.6998)
  line L628 (-6.7692, 123.6998) -> (-6.7692, 120.6998)
  line L629 (-11.9654, 120.6998) -> (-11.9654, 123.6998)
  line L630 (-11.9654, 123.6998) -> (-9.3673, 125.1998)
  line L631 (-9.3673, 125.1998) -> (-6.7692, 123.6998)
  line L632 (-6.7692, 120.6998) -> (-9.3673, 119.1998)
  line L633 (-2.6712, 119.1998) -> (-5.2692, 120.6998)
  line L634 (-0.0731, 123.6998) -> (-0.0731, 120.6998)
  line L635 (-5.2692, 120.6998) -> (-5.2692, 123.6998)
  line L636 (-5.2692, 123.6998) -> (-2.6712, 125.1998)
  line L637 (-1.35, 124.437) -> (-0.0731, 123.6998)
  line L638 (-0.0731, 120.6998) -> (-1.35, 119.9625)
  line L639 (-38.75, 120.6998) -> (-38.75, 123.6998)
  line L640 (-38.75, 123.6998) -> (-36.1519, 125.1998)
  line L641 (-36.1519, 119.1998) -> (-38.75, 120.6998)
  line L642 (-33.5538, 123.6998) -> (-33.5538, 120.6998)
  line L643 (-36.1519, 125.1998) -> (-33.5538, 123.6998)
  line L644 (-33.5538, 120.6998) -> (-36.1519, 119.1998)
  line L645 (-30.2058, 129.6998) -> (-30.2058, 126.6998)
  line L646 (-30.2058, 126.6998) -> (-32.8038, 125.1998)
  line L647 (-32.8038, 125.1998) -> (-35.4019, 126.6998)
  line L648 (-35.4019, 126.6998) -> (-35.4019, 129.6998)
  line L649 (-35.4019, 129.6998) -> (-32.8038, 131.1998)
  line L650 (-32.8038, 131.1998) -> (-30.2058, 129.6998)
  line L651 (-28.7058, 126.6998) -> (-28.7058, 129.6998)
  line L652 (-28.7058, 129.6998) -> (-26.1077, 131.1998)
  line L653 (-26.1077, 131.1998) -> (-23.5096, 129.6998)
  line L654 (-23.5096, 129.6998) -> (-23.5096, 126.6998)
  line L655 (-23.5096, 126.6998) -> (-26.1077, 125.1998)
  line L656 (-26.1077, 125.1998) -> (-28.7058, 126.6998)
  line L657 (-19.4115, 125.1998) -> (-22.0096, 126.6998)
  line L658 (-16.8135, 129.6998) -> (-16.8135, 126.6998)
  line L659 (-22.0096, 126.6998) -> (-22.0096, 129.6998)
  line L660 (-22.0096, 129.6998) -> (-19.4115, 131.1998)
  line L661 (-19.4115, 131.1998) -> (-16.8135, 129.6998)
  line L662 (-16.8135, 126.6998) -> (-19.4115, 125.1998)
  line L663 (-12.7154, 125.1998) -> (-15.3135, 126.6998)
  line L664 (-10.1173, 129.6998) -> (-10.1173, 126.6998)
  line L665 (-15.3135, 126.6998) -> (-15.3135, 129.6998)
  line L666 (-15.3135, 129.6998) -> (-12.7154, 131.1998)
  line L667 (-12.7154, 131.1998) -> (-10.1173, 129.6998)
  line L668 (-10.1173, 126.6998) -> (-12.7154, 125.1998)
  line L669 (-6.0192, 125.1998) -> (-8.6173, 126.6998)
  line L670 (-3.4212, 129.6998) -> (-3.4212, 126.6998)
  line L671 (-8.6173, 126.6998) -> (-8.6173, 129.6998)
  line L672 (-8.6173, 129.6998) -> (-6.0192, 131.1998)
  line L673 (-6.0192, 131.1998) -> (-3.4212, 129.6998)
  line L674 (-3.4212, 126.6998) -> (-6.0192, 125.1998)
  line L675 (-42.0981, 126.6998) -> (-42.0981, 129.6998)
  line L676 (-42.0981, 129.6998) -> (-39.5, 131.1998)
  line L677 (-39.5, 125.1998) -> (-42.0981, 126.6998)
  line L678 (-36.9019, 129.6998) -> (-36.9019, 126.6998)
  line L679 (-39.5, 131.1998) -> (-36.9019, 129.6998)
  line L680 (-36.9019, 126.6998) -> (-39.5, 125.1998)
  line L681 (-26.8577, 135.6998) -> (-26.8577, 132.6998)
  line L682 (-26.8577, 132.6998) -> (-29.4558, 131.1998)
  line L683 (-29.4558, 131.1998) -> (-32.0538, 132.6998)
  line L684 (-32.0538, 132.6998) -> (-32.0538, 135.6998)
  line L685 (-32.0538, 135.6998) -> (-29.4558, 137.1998)
  line L686 (-29.4558, 137.1998) -> (-26.8577, 135.6998)
  line L687 (-25.3577, 132.6998) -> (-25.3577, 135.6998)
  line L688 (-25.3577, 135.6998) -> (-22.7596, 137.1998)
  line L689 (-22.7596, 137.1998) -> (-20.1615, 135.6998)
  line L690 (-20.1615, 135.6998) -> (-20.1615, 132.6998)
  line L691 (-20.1615, 132.6998) -> (-22.7596, 131.1998)
  line L692 (-22.7596, 131.1998) -> (-25.3577, 132.6998)
  line L693 (-16.0635, 131.1998) -> (-18.6615, 132.6998)
  line L694 (-13.4654, 135.6998) -> (-13.4654, 132.6998)
  line L695 (-18.6615, 132.6998) -> (-18.6615, 135.6998)
  line L696 (-18.6615, 135.6998) -> (-16.0635, 137.1998)
  line L697 (-16.0635, 137.1998) -> (-13.4654, 135.6998)
  line L698 (-13.4654, 132.6998) -> (-16.0635, 131.1998)
  line L699 (-9.3673, 131.1998) -> (-11.9654, 132.6998)
  line L700 (-6.7692, 135.6998) -> (-6.7692, 132.6998)
  line L701 (-11.9654, 132.6998) -> (-11.9654, 135.6998)
  line L702 (-11.9654, 135.6998) -> (-9.3673, 137.1998)
  line L703 (-9.3673, 137.1998) -> (-6.7692, 135.6998)
  line L704 (-6.7692, 132.6998) -> (-9.3673, 131.1998)
  line L705 (-2.6712, 131.1998) -> (-5.2692, 132.6998)
  line L706 (-0.0731, 135.6998) -> (-0.0731, 132.6998)
  line L707 (-5.2692, 132.6998) -> (-5.2692, 135.6998)
  line L708 (-5.2692, 135.6998) -> (-2.6712, 137.1998)
  line L709 (-1.35, 136.437) -> (-0.0731, 135.6998)
  line L710 (-0.0731, 132.6998) -> (-1.35, 131.9625)
  line L711 (-38.75, 132.6998) -> (-38.75, 135.6998)
  line L712 (-38.75, 135.6998) -> (-36.1519, 137.1998)
  line L713 (-36.1519, 131.1998) -> (-38.75, 132.6998)
  line L714 (-33.5538, 135.6998) -> (-33.5538, 132.6998)
  line L715 (-36.1519, 137.1998) -> (-33.5538, 135.6998)
  line L716 (-33.5538, 132.6998) -> (-36.1519, 131.1998)
  line L717 (-30.2924, 141.6498) -> (-30.2924, 138.7498)
  line L718 (-30.2924, 138.7498) -> (-32.8038, 137.2998)
  line L719 (-32.8038, 137.2998) -> (-35.3153, 138.7498)
  line L720 (-35.3153, 138.7498) -> (-35.3153, 141.6498)
  line L721 (-35.3153, 141.6498) -> (-34.1025, 142.35)
  line L722 (-31.5052, 142.35) -> (-30.2924, 141.6498)
  line L723 (-28.6192, 138.7498) -> (-28.6192, 141.6498)
  line L724 (-28.6192, 141.6498) -> (-27.4063, 142.35)
  line L725 (-24.8091, 142.35) -> (-23.5962, 141.6498)
  line L726 (-23.5962, 141.6498) -> (-23.5962, 138.7498)
  line L727 (-23.5962, 138.7498) -> (-26.1077, 137.2998)
  line L728 (-26.1077, 137.2998) -> (-28.6192, 138.7498)
  line L729 (-19.4115, 137.2998) -> (-21.923, 138.7498)
  line L730 (-16.9001, 141.6498) -> (-16.9001, 138.7498)
  line L731 (-21.923, 138.7498) -> (-21.923, 141.6498)
  line L732 (-21.923, 141.6498) -> (-20.7102, 142.35)
  line L733 (-18.1129, 142.35) -> (-16.9001, 141.6498)
  line L734 (-16.9001, 138.7498) -> (-19.4115, 137.2998)
  line L735 (-12.7154, 137.2998) -> (-15.2269, 138.7498)
  line L736 (-10.2039, 141.6498) -> (-10.2039, 138.7498)
  line L737 (-15.2269, 138.7498) -> (-15.2269, 141.6498)
  line L738 (-15.2269, 141.6498) -> (-14.014, 142.35)
  line L739 (-11.4168, 142.35) -> (-10.2039, 141.6498)
  line L740 (-10.2039, 138.7498) -> (-12.7154, 137.2998)
  line L741 (-6.0192, 137.2998) -> (-8.5307, 138.7498)
  line L742 (-3.5078, 141.6498) -> (-3.5078, 138.7498)
  line L743 (-8.5307, 138.7498) -> (-8.5307, 141.6498)
  line L744 (-8.5307, 141.6498) -> (-7.3179, 142.35)
  line L745 (-4.7206, 142.35) -> (-3.5078, 141.6498)
  line L746 (-3.5078, 138.7498) -> (-6.0192, 137.2998)
  line L747 (-42.0115, 138.7498) -> (-42.0115, 141.6498)
  line L748 (-42.0115, 141.6498) -> (-40.65, 142.4358)
  line L749 (-39.5, 137.2998) -> (-42.0115, 138.7498)
  line L750 (-36.9885, 141.6498) -> (-36.9885, 138.7498)
  line L751 (-38.2014, 142.35) -> (-36.9885, 141.6498)
  line L752 (-36.9885, 138.7498) -> (-39.5, 137.2998)
  line L753 (-2.5841, 23.25) -> (-5.1822, 24.75)
  line L754 (-6.6822, 24.75) -> (-9.2803, 23.25)
  line L755 (0.0139, 27.75) -> (0.0139, 24.75)
  line L756 (-5.1822, 24.75) -> (-5.1822, 27.75)
  line L757 (-1.35, 28.5375) -> (0.0139, 27.75)
  line L758 (-5.1822, 27.75) -> (-2.5841, 29.25)
  line L759 (-9.2803, 29.25) -> (-6.6822, 27.75)
  line L760 (0.0139, 24.75) -> (-1.35, 23.9625)
  line L761 (-6.6822, 27.75) -> (-6.6822, 24.75)
  line L762 (-22.6726, 23.25) -> (-25.2707, 24.75)
  line L763 (-25.2707, 24.75) -> (-25.2707, 27.75)
  line L764 (-25.2707, 27.75) -> (-22.6726, 29.25)
  line L765 (-20.0745, 24.75) -> (-22.6726, 23.25)
  line L766 (-22.6726, 29.25) -> (-20.0745, 27.75)
  line L767 (-20.0745, 27.75) -> (-20.0745, 24.75)
  line L768 (-18.5745, 24.75) -> (-18.5745, 27.75)
  line L769 (-13.3784, 24.75) -> (-15.9764, 23.25)
  line L770 (-18.5745, 27.75) -> (-15.9764, 29.25)
  line L771 (-13.3784, 27.75) -> (-13.3784, 24.75)
  line L772 (-15.9764, 29.25) -> (-13.3784, 27.75)
  line L773 (-11.8784, 24.75) -> (-11.8784, 27.75)
  line L774 (-9.2803, 23.25) -> (-11.8784, 24.75)
  line L775 (-11.8784, 27.75) -> (-9.2803, 29.25)
  line L776 (-15.9764, 23.25) -> (-18.5745, 24.75)
  line L777 (-29.3688, 23.25) -> (-31.9668, 24.75)
  line L778 (-33.4668, 24.75) -> (-36.0649, 23.25)
  line L779 (-26.7707, 24.75) -> (-29.3688, 23.25)
  line L780 (-36.0649, 23.25) -> (-38.663, 24.75)
  line L781 (-33.4668, 27.75) -> (-33.4668, 24.75)
  line L782 (-38.663, 24.75) -> (-38.663, 27.75)
  line L783 (-38.663, 27.75) -> (-36.0649, 29.25)
  line L784 (-36.0649, 29.25) -> (-33.4668, 27.75)
  line L785 (-31.9668, 24.75) -> (-31.9668, 27.75)
  line L786 (-26.7707, 27.75) -> (-26.7707, 24.75)
  line L787 (-29.3688, 29.25) -> (-26.7707, 27.75)
  line L788 (-31.9668, 27.75) -> (-29.3688, 29.25)
  line L789 (-2.6712, 11.25) -> (-5.2692, 12.75)
  line L790 (-6.7692, 12.75) -> (-9.3673, 11.25)
  line L791 (-0.0731, 15.75) -> (-0.0731, 12.75)
  line L792 (-5.2692, 12.75) -> (-5.2692, 15.75)
  line L793 (-1.35, 16.4872) -> (-0.0731, 15.75)
  line L794 (-5.2692, 15.75) -> (-2.6712, 17.25)
  line L795 (-9.3673, 17.25) -> (-6.7692, 15.75)
  line L796 (-0.0731, 12.75) -> (-1.35, 12.0128)
  line L797 (-6.7692, 15.75) -> (-6.7692, 12.75)
  line L798 (-22.7596, 11.25) -> (-25.3577, 12.75)
  line L799 (-25.3577, 12.75) -> (-25.3577, 15.75)
  line L800 (-25.3577, 15.75) -> (-22.7596, 17.25)
  line L801 (-20.1615, 12.75) -> (-22.7596, 11.25)
  line L802 (-22.7596, 17.25) -> (-20.1615, 15.75)
  line L803 (-20.1615, 15.75) -> (-20.1615, 12.75)
  line L804 (-18.6615, 12.75) -> (-18.6615, 15.75)
  line L805 (-13.4654, 12.75) -> (-16.0635, 11.25)
  line L806 (-18.6615, 15.75) -> (-16.0635, 17.25)
  line L807 (-13.4654, 15.75) -> (-13.4654, 12.75)
  line L808 (-16.0635, 17.25) -> (-13.4654, 15.75)
  line L809 (-11.9654, 12.75) -> (-11.9654, 15.75)
  line L810 (-9.3673, 11.25) -> (-11.9654, 12.75)
  line L811 (-11.9654, 15.75) -> (-9.3673, 17.25)
  line L812 (-16.0635, 11.25) -> (-18.6615, 12.75)
  line L813 (-29.4558, 11.25) -> (-32.0538, 12.75)
  line L814 (-33.5538, 12.75) -> (-36.1519, 11.25)
  line L815 (-26.8577, 12.75) -> (-29.4558, 11.25)
  line L816 (-36.1519, 11.25) -> (-38.75, 12.75)
  line L817 (-33.5538, 15.75) -> (-33.5538, 12.75)
  line L818 (-38.75, 12.75) -> (-38.75, 15.75)
  line L819 (-38.75, 15.75) -> (-36.1519, 17.25)
  line L820 (-36.1519, 17.25) -> (-33.5538, 15.75)
  line L821 (-32.0538, 12.75) -> (-32.0538, 15.75)
  line L822 (-26.8577, 15.75) -> (-26.8577, 12.75)
  line L823 (-29.4558, 17.25) -> (-26.8577, 15.75)
  line L824 (-32.0538, 15.75) -> (-29.4558, 17.25)
  point P0 (0, 0)
  point P1 (-36.1519, 14.25)
  point P2 (-32.8038, 20.25)
  point P3 (-29.4558, 14.25)
  point P4 (-26.1077, 20.25)
  point P5 (-19.4115, 20.25)
  point P6 (-12.7154, 20.25)
  point P7 (-6.0192, 20.25)
  point P8 (-39.5, 20.25)
  point P9 (-23.4226, 18.6998)
  point P10 (-32.8038, 32.1998)
  point P11 (-26.1077, 32.1998)
  point P12 (-19.4115, 32.1998)
  point P13 (-12.7154, 32.1998)
  point P14 (-6.0192, 32.1998)
  point P15 (-39.5, 32.1998)
  point P16 (-32.8038, 35.1998)
  point P17 (-29.4558, 38.1998)
  point P18 (-26.1077, 35.1998)
  point P19 (-22.7596, 38.1998)
  point P20 (-16.0635, 38.1998)
  point P21 (-9.3673, 38.1998)
  point P22 (-2.6712, 38.1998)
  point P23 (-36.1519, 38.1998)
  point P24 (-36.1519, 41.1998)
  point P25 (-32.8038, 44.1998)
  point P26 (-29.4558, 41.1998)
  point P27 (-26.8577, 36.6998)
  point P28 (-26.1077, 44.1998)
  point P29 (-19.4115, 44.1998)
  point P30 (-12.7154, 44.1998)
  point P31 (-6.0192, 44.1998)
  point P32 (-39.5, 44.1998)
  point P33 (-32.8038, 47.1998)
  point P34 (-29.4558, 50.1998)
  point P35 (-26.1077, 47.1998)
  point P36 (-22.7596, 50.1998)
  point P37 (-16.0635, 50.1998)
  point P38 (-9.3673, 50.1998)
  point P39 (-2.6712, 50.1998)
  point P40 (-36.1519, 50.1998)
  point P41 (-36.1519, 53.1998)
  point P42 (-32.8038, 56.1998)
  point P43 (-29.4558, 53.1998)
  point P44 (-26.8577, 48.6998)
  point P45 (-26.1077, 56.1998)
  point P46 (-19.4115, 56.1998)
  point P47 (-12.7154, 56.1998)
  point P48 (-6.0192, 56.1998)
  point P49 (-39.5, 56.1998)
  point P50 (-32.8038, 59.1998)
  point P51 (-29.4558, 62.1998)
  point P52 (-26.1077, 59.1998)
  point P53 (-22.7596, 62.1998)
  point P54 (-16.0635, 62.1998)
  point P55 (-9.3673, 62.1998)
  point P56 (-2.6712, 62.1998)
  point P57 (-36.1519, 62.1998)
  point P58 (-36.1519, 65.1998)
  point P59 (-32.8038, 68.1998)
  point P60 (-29.4558, 65.1998)
  point P61 (-26.8577, 60.6998)
  point P62 (-26.1077, 68.1998)
  point P63 (-19.4115, 68.1998)
  point P64 (-12.7154, 68.1998)
  point P65 (-6.0192, 68.1998)
  point P66 (-39.5, 68.1998)
  point P67 (-32.8038, 71.1998)
  point P68 (-29.4558, 74.1998)
  point P69 (-26.1077, 71.1998)
  point P70 (-22.7596, 74.1998)
  point P71 (-16.0635, 74.1998)
  point P72 (-9.3673, 74.1998)
  point P73 (-2.6712, 74.1998)
  point P74 (-36.1519, 74.1998)
  point P75 (-36.1519, 77.1998)
  point P76 (-32.8038, 80.1998)
  point P77 (-29.4558, 77.1998)
  point P78 (-26.8577, 72.6998)
  point P79 (-26.1077, 80.1998)
  point P80 (-19.4115, 80.1998)
  point P81 (-12.7154, 80.1998)
  point P82 (-6.0192, 80.1998)
  point P83 (-39.5, 80.1998)
  point P84 (-32.8038, 83.1998)
  point P85 (-29.4558, 86.1998)
  point P86 (-26.1077, 83.1998)
  point P87 (-22.7596, 86.1998)
  point P88 (-16.0635, 86.1998)
  point P89 (-9.3673, 86.1998)
  point P90 (-2.6712, 86.1998)
  point P91 (-36.1519, 86.1998)
  point P92 (-36.1519, 89.1998)
  point P93 (-32.8038, 92.1998)
  point P94 (-29.4558, 89.1998)
  point P95 (-26.8577, 84.6998)
  point P96 (-26.1077, 92.1998)
  point P97 (-19.4115, 92.1998)
  point P98 (-12.7154, 92.1998)
  point P99 (-6.0192, 92.1998)
  point P100 (-39.5, 92.1998)
  point P101 (-32.8038, 95.1998)
  point P102 (-29.4558, 98.1998)
  point P103 (-26.1077, 95.1998)
  point P104 (-22.7596, 98.1998)
  point P105 (-16.0635, 98.1998)
  point P106 (-9.3673, 98.1998)
  point P107 (-2.6712, 98.1998)
  point P108 (-36.1519, 98.1998)
  point P109 (-36.1519, 101.1998)
  point P110 (-32.8038, 104.1998)
  point P111 (-29.4558, 101.1998)
  point P112 (-26.8577, 96.6998)
  point P113 (-26.1077, 104.1998)
  point P114 (-19.4115, 104.1998)
  point P115 (-12.7154, 104.1998)
  point P116 (-6.0192, 104.1998)
  point P117 (-39.5, 104.1998)
  point P118 (-32.8038, 107.1998)
  point P119 (-29.4558, 110.1998)
  point P120 (-26.1077, 107.1998)
  point P121 (-22.7596, 110.1998)
  point P122 (-16.0635, 110.1998)
  point P123 (-9.3673, 110.1998)
  point P124 (-2.6712, 110.1998)
  point P125 (-36.1519, 110.1998)
  point P126 (-36.1519, 113.1998)
  point P127 (-32.8038, 116.1998)
  point P128 (-29.4558, 113.1998)
  point P129 (-26.8577, 108.6998)
  point P130 (-26.1077, 116.1998)
  point P131 (-19.4115, 116.1998)
  point P132 (-12.7154, 116.1998)
  point P133 (-6.0192, 116.1998)
  point P134 (-39.5, 116.1998)
  point P135 (-32.8038, 119.1998)
  point P136 (-29.4558, 122.1998)
  point P137 (-26.1077, 119.1998)
  point P138 (-22.7596, 122.1998)
  point P139 (-16.0635, 122.1998)
  point P140 (-9.3673, 122.1998)
  point P141 (-2.6712, 122.1998)
  point P142 (-36.1519, 122.1998)
  point P143 (-36.1519, 125.1998)
  point P144 (-32.8038, 128.1998)
  point P145 (-29.4558, 125.1998)
  point P146 (-26.8577, 120.6998)
  point P147 (-26.1077, 128.1998)
  point P148 (-19.4115, 128.1998)
  point P149 (-12.7154, 128.1998)
  point P150 (-6.0192, 128.1998)
  point P151 (-39.5, 128.1998)
  point P152 (-32.8038, 131.1998)
  point P153 (-29.4558, 134.1998)
  point P154 (-26.1077, 131.1998)